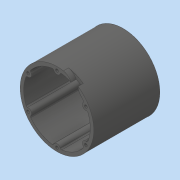
# Autodesk Inventor part: Spool
Saved by Autodesk Inventor 2017 (Build 210142000, 142)
## iProperties
Created: 2016-11-06
Part Number: Spool
Material: ABS Plastic
Document SubType Name: Modeling
Designer: techn
Density: 1.06 g/cm^3
Appearance: Gray
Author: techn
Autodesk Inventor part; units mm, degrees
ref_plane "YZ Plane" through (0, 0, 0) normal (1, 0, 0) x (0, 1, 0)
ref_plane "XZ Plane" through (0, 0, 0) normal (0, 1, 0) x (-1, 0, 0)
ref_plane "XY Plane" through (0, 0, 0) normal (0, 0, 1) x (1, 0, 0)
sketch "Sketch1" plane through (0, 0, 0) normal (0, 0, 1) x (1, 0, 0)
  circle A0 centre (0, 0) radius 33.655
  circle A1 centre (0, 0) radius 30.48
  dimension "d0" = 67.31
  dimension "d1" = 60.96
  constraints: 2 centre point, 2 coincident
  measures "d0" diameter of A0
  measures "d1" diameter of A1
extrude "Extrusion1" add sketch "Sketch1" along normal blind 60.325
sketch "Sketch3" plane through (0, 0, 60.325) normal (0, 0, 1) x (1, 0, 0)
  line L0 (0, 0) -> (0, 30.48)
  circle A0 centre (0, 30.48) radius 1.27
  circle A1 centre (0, 30.48) radius 3.175
  circle A2 centre (-26.3965, 15.24) radius 3.175
  circle A3 centre (-26.3965, 15.24) radius 1.27
  circle A4 centre (-26.3965, -15.24) radius 3.175
  circle A5 centre (-26.3965, -15.24) radius 1.27
  circle A6 centre (0, -30.48) radius 3.175
  circle A7 centre (0, -30.48) radius 1.27
  circle A8 centre (26.3965, -15.24) radius 3.175
  circle A9 centre (26.3965, -15.24) radius 1.27
  circle A10 centre (26.3965, 15.24) radius 3.175
  circle A11 centre (26.3965, 15.24) radius 1.27
  dimension "d4" = 30.48
  dimension "d5" = 2.54
  dimension "d6" = 6.35
  dimension "d9" = 360
  constraints: 12 centre point, 7 coincident, 2 end point, 1 vertical, 25 other
  measures "d4" distance of L0.start L0.end
  measures "d5" diameter of A0
  measures "d6" diameter of A1
extrude "Extrusion2" add sketch "Sketch3" against normal up to surface (60.325 mm away)
extrude "Extrusion3" cut sketch "Sketch3" against normal up to surface (60.325 mm away) contours A0 | A3 | A5 | A7 | A9 | A11
sketch "Sketch4" plane through (0, 0, 60.325) normal (0, 0, 1) x (1, 0, 0)
  circle A0 centre (26.3965, -15.24) radius 1.27 projected
  arc A1 (27.8386, -12.4114) -> (24.6679, -17.9032) centre (26.3965, -15.24) ccw projected
  arc A2 (3.1707, -30.3146) -> (24.6679, -17.9032) centre (0, 0) ccw projected
  arc A3 (3.1707, -30.3146) -> (-3.1707, -30.3146) centre (0, -30.48) ccw projected
  arc A4 (-24.6679, -17.9032) -> (-3.1707, -30.3146) centre (0, 0) ccw projected
  arc A5 (-24.6679, -17.9032) -> (-27.8386, -12.4114) centre (-26.3965, -15.24) ccw projected
  arc A6 (-27.8386, 12.4114) -> (-27.8386, -12.4114) centre (0, 0) ccw projected
  arc A7 (-27.8386, 12.4114) -> (-24.6679, 17.9032) centre (-26.3965, 15.24) ccw projected
  arc A8 (-3.1707, 30.3146) -> (-24.6679, 17.9032) centre (0, 0) ccw projected
  arc A9 (-3.1707, 30.3146) -> (3.1707, 30.3146) centre (0, 30.48) ccw projected
  arc A10 (24.6679, 17.9032) -> (3.1707, 30.3146) centre (0, 0) ccw projected
  arc A11 (24.6679, 17.9032) -> (27.8386, 12.4114) centre (26.3965, 15.24) ccw projected
  arc A12 (27.8386, -12.4114) -> (27.8386, 12.4114) centre (0, 0) ccw projected
  circle A13 centre (0, -30.48) radius 1.27 projected
  circle A14 centre (26.3965, 15.24) radius 1.27 projected
  circle A15 centre (-26.3965, 15.24) radius 1.27 projected
  circle A16 centre (0, 30.48) radius 1.27 projected
  circle A17 centre (0, 0) radius 33.655 projected
  circle A18 centre (-26.3965, -15.24) radius 1.27 projected
  line L0 (0, 0) -> (19.3037, 27.5686)
  circle A19 centre (0, 0) radius 33.655 projected
  line L1 (0, 0) -> (33.655, 0) construction
  line L2 (0, 0) -> (14.2232, 30.5018)
  line L3 (0, 0) -> (33.655, 0) construction
  arc A20 (19.3037, 27.5686) -> (14.2232, 30.5018) centre (0, 0) ccw
  arc A21 (24.6679, 17.9032) -> (3.1707, 30.3146) centre (0, 0) ccw projected
  arc A22 (17.4826, 24.9678) -> (12.8814, 27.6243) centre (0, 0) ccw
  dimension "d15" = 55
  dimension "d16" = 65
  constraints: 8 end point, 8 point on circle, 2 centre point, 2 equal length, 2 horizontal, 2 point on line
  measures "d15" angle of L1 L0
  measures "d16" angle of L3 L2
extrude "Extrusion4" cut sketch "Sketch4" against normal blind 4.699 contours A10 L2 A17 L0
fillet "Fillet1" radius 9.525 2 edges at (14.2232, 30.5018, 57.9755) (17.4826, 24.9678, 57.9755)
fillet "Fillet2" radius 1.27 12 edges at (-27.8386, -12.4114, 30.1625) (-24.6679, -17.9032, 30.1625) (-27.8386, 12.4114, 30.1625) (-24.6679, 17.9032, 30.1625) (3.1707, 30.3146, 30.1625) (-3.1707, 30.3146, 30.1625) (24.6679, -17.9032, 30.1625) (27.8386, -12.4114, 30.1625) (27.8386, 12.4114, 30.1625) (24.6679, 17.9032, 30.1625) (-3.1707, -30.3146, 30.1625) (3.1707, -30.3146, 30.1625)
body "Solid1"
